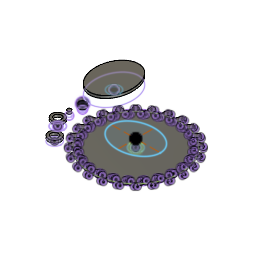
Duck Machine Gear 1 (Autodesk Fusion 360 design; units mm, degrees)
part number: 2026-02-17-17-01-41-865
Autodesk Fusion 360 part; units mm, degrees
(part 1 of 6)
sketch "Base Circle" plane through (0, 0, 0) normal (0, 0, 1) x (1, 0, 0)
  circle A0 centre (0, 0) radius 65.058
  circle A1 centre (0, 0) radius 2.45
extrude "Extrude3" add sketch "Base Circle" along normal blind 4.2 makes body 1
sketch "Gear Tooth" plane through (0, 0, 0) normal (0, 0, 1) x (1, 0, 0)
  spline S0 degree 5 poles (67.4396, -5.4307) (67.47, -5.4332) (67.531, -5.4373) (67.6225, -5.4412) (67.7446, -5.442) (67.8973, -5.437) (68.0502, -5.4277) (68.2031, -5.4157) (68.3561, -5.4023) (68.5091, -5.3879) (68.6621, -5.3725) (68.815, -5.3558) (68.968, -5.3372) (69.1209, -5.3166) (69.2738, -5.2939) (69.4267, -5.2693) (69.5795, -5.243) (69.7323, -5.2153) (69.885, -5.1864) (70.0377, -5.1565) (70.1903, -5.1253) (70.3428, -5.093) (70.4953, -5.0595) (70.6477, -5.0246) (70.8, -4.9885) (70.9522, -4.9511) (71.1044, -4.9126) (71.2565, -4.873) (71.4084, -4.8323) (71.5603, -4.7906) (71.7121, -4.7478) (71.8638, -4.704) (72.0153, -4.6592) (72.1668, -4.6134) (72.3182, -4.5666) (72.4695, -4.5187) (72.6206, -4.4699) (72.7716, -4.4202) (72.9226, -4.3695) (73.0734, -4.3179) (73.224, -4.2653) (73.3746, -4.2119) (73.525, -4.1576) (73.6753, -4.1023) (73.8255, -4.0462) (73.9756, -3.9892) (74.1255, -3.9313) (74.2752, -3.8726) (74.4249, -3.8131) (74.5744, -3.7527) (74.7237, -3.6914) (74.873, -3.6294) (75.022, -3.5665) (75.171, -3.5028) (75.3197, -3.4383) (75.4684, -3.373) (75.6168, -3.3069) (75.7652, -3.2401) (75.9133, -3.1724) (76.0614, -3.104) (76.2092, -3.0348) (76.3569, -2.9648) (76.5044, -2.8941) (76.6518, -2.8227) (76.799, -2.7505) (76.946, -2.6775) (77.0929, -2.6038) (77.2396, -2.5294) (77.3861, -2.4543) (77.5325, -2.3784) (77.6787, -2.3019) (77.7955, -2.24) (77.883, -2.1933) (77.9413, -2.1621) (77.9705, -2.1464) knots 0 0 0 0 0 0 0.01428571 0.02857143 0.04285714 0.05714286 0.07142857 0.08571429 0.1 0.11428571 0.12857143 0.14285714 0.15714286 0.17142857 0.18571429 0.2 0.21428571 0.22857143 0.24285714 0.25714286 0.27142857 0.28571429 0.3 0.31428571 0.32857143 0.34285714 0.35714286 0.37142857 0.38571429 0.4 0.41428571 0.42857143 0.44285714 0.45714286 0.47142857 0.48571429 0.5 0.51428571 0.52857143 0.54285714 0.55714286 0.57142857 0.58571429 0.6 0.61428571 0.62857143 0.64285714 0.65714286 0.67142857 0.68571429 0.7 0.71428571 0.72857143 0.74285714 0.75714286 0.77142857 0.78571429 0.8 0.81428571 0.82857143 0.84285714 0.85714286 0.87142857 0.88571429 0.9 0.91428571 0.92857143 0.94285714 0.95714286 0.97142857 0.98571429 1 1 1 1 1 1
  spline S1 degree 5 poles (67.4396, 5.4307) (67.47, 5.4332) (67.531, 5.4373) (67.6225, 5.4412) (67.7446, 5.442) (67.8973, 5.437) (68.0502, 5.4277) (68.2031, 5.4157) (68.3561, 5.4023) (68.5091, 5.3879) (68.6621, 5.3725) (68.815, 5.3558) (68.968, 5.3372) (69.1209, 5.3166) (69.2738, 5.2939) (69.4267, 5.2693) (69.5795, 5.243) (69.7323, 5.2153) (69.885, 5.1864) (70.0377, 5.1565) (70.1903, 5.1253) (70.3428, 5.093) (70.4953, 5.0595) (70.6477, 5.0246) (70.8, 4.9885) (70.9522, 4.9511) (71.1044, 4.9126) (71.2565, 4.873) (71.4084, 4.8323) (71.5603, 4.7906) (71.7121, 4.7478) (71.8638, 4.704) (72.0153, 4.6592) (72.1668, 4.6134) (72.3182, 4.5666) (72.4695, 4.5187) (72.6206, 4.4699) (72.7716, 4.4202) (72.9226, 4.3695) (73.0734, 4.3179) (73.224, 4.2653) (73.3746, 4.2119) (73.525, 4.1576) (73.6753, 4.1023) (73.8255, 4.0462) (73.9756, 3.9892) (74.1255, 3.9313) (74.2752, 3.8726) (74.4249, 3.8131) (74.5744, 3.7527) (74.7237, 3.6914) (74.873, 3.6294) (75.022, 3.5665) (75.171, 3.5028) (75.3197, 3.4383) (75.4684, 3.373) (75.6168, 3.3069) (75.7652, 3.2401) (75.9133, 3.1724) (76.0614, 3.104) (76.2092, 3.0348) (76.3569, 2.9648) (76.5044, 2.8941) (76.6518, 2.8227) (76.799, 2.7505) (76.946, 2.6775) (77.0929, 2.6038) (77.2396, 2.5294) (77.3861, 2.4543) (77.5325, 2.3784) (77.6787, 2.3019) (77.7955, 2.24) (77.883, 2.1933) (77.9413, 2.1621) (77.9705, 2.1464) knots 0 0 0 0 0 0 0.01428571 0.02857143 0.04285714 0.05714286 0.07142857 0.08571429 0.1 0.11428571 0.12857143 0.14285714 0.15714286 0.17142857 0.18571429 0.2 0.21428571 0.22857143 0.24285714 0.25714286 0.27142857 0.28571429 0.3 0.31428571 0.32857143 0.34285714 0.35714286 0.37142857 0.38571429 0.4 0.41428571 0.42857143 0.44285714 0.45714286 0.47142857 0.48571429 0.5 0.51428571 0.52857143 0.54285714 0.55714286 0.57142857 0.58571429 0.6 0.61428571 0.62857143 0.64285714 0.65714286 0.67142857 0.68571429 0.7 0.71428571 0.72857143 0.74285714 0.75714286 0.77142857 0.78571429 0.8 0.81428571 0.82857143 0.84285714 0.85714286 0.87142857 0.88571429 0.9 0.91428571 0.92857143 0.94285714 0.95714286 0.97142857 0.98571429 1 1 1 1 1 1
  arc A0 (77.9705, -2.1464) -> (77.9705, 2.1464) centre (0, 0) ccw
  line L0 (64.8381, -5.2213) -> (67.4396, -5.4307)
  line L1 (64.8381, 5.2213) -> (67.4396, 5.4307)
  line L2 (64.8381, -5.2213) -> (64.8381, 5.2213)
  point P0 (68.1817, -5.4171)
  point P1 (68.9286, -5.3417)
  point P2 (69.6784, -5.2249)
  point P3 (70.4303, -5.0736)
  point P4 (71.1836, -4.8918)
  point P5 (71.938, -4.682)
  point P6 (72.6931, -4.4459)
  point P7 (73.4485, -4.1851)
  point P8 (74.2039, -3.9005)
  point P9 (74.959, -3.5929)
  point P10 (75.7135, -3.2632)
  point P11 (76.4671, -2.9119)
  point P12 (77.2195, -2.5395)
  point P13 (68.1817, 5.4171)
  point P14 (68.9286, 5.3417)
  point P15 (69.6784, 5.2249)
  point P16 (70.4303, 5.0736)
  point P17 (71.1836, 4.8918)
  point P18 (71.938, 4.682)
  point P19 (72.6931, 4.4459)
  point P20 (73.4485, 4.1851)
  point P21 (74.2039, 3.9005)
  point P22 (74.959, 3.5929)
  point P23 (75.7135, 3.2632)
  point P24 (76.4671, 2.9119)
  point P25 (77.2195, 2.5395)
extrude "Extrude4" add sketch "Gear Tooth" along normal blind 4.2 bodies 1
fillet "Fillet2" radius 2 2 edges at (64.8481, -5.2221, 2.1) (64.8481, 5.2221, 2.1) on bodies 1
pattern_circular "C-Pattern2" count 24 over 360 about axis through (0, 0, 0) along (0, 0, 1) of "Extrude4", "Fillet2"
sketch "Diametrial Pitch Circle" plane through (0, 0, 0) normal (0, 0, 1) x (1, 0, 0)
  circle A0 centre (0, 0) radius 72 construction
sketch "Spacer and Cap" plane through (0, 0, 4.2) normal (0, 0, 1) x (-1, 0, 0)
  arc A0 (-64.3117, 9.8261) -> (-64.6635, 7.1538) centre (0, 0) ccw
  arc A1 (-66.8119, 5.3802) -> (-64.6635, 7.1538) centre (-66.6514, 7.3737) ccw
  line L0 (-66.8119, 5.3802) -> (-67.4396, 5.4307)
  spline S0 degree 5 poles (-67.4396, 5.4307) (-67.47, 5.4332) (-67.531, 5.4373) (-67.6225, 5.4412) (-67.7446, 5.442) (-67.8973, 5.437) (-68.0502, 5.4277) (-68.2031, 5.4157) (-68.3561, 5.4023) (-68.5091, 5.3879) (-68.6621, 5.3725) (-68.815, 5.3558) (-68.968, 5.3372) (-69.1209, 5.3166) (-69.2738, 5.2939) (-69.4267, 5.2693) (-69.5795, 5.243) (-69.7323, 5.2153) (-69.885, 5.1864) (-70.0377, 5.1565) (-70.1903, 5.1253) (-70.3428, 5.093) (-70.4953, 5.0595) (-70.6477, 5.0246) (-70.8, 4.9885) (-70.9522, 4.9511) (-71.1044, 4.9126) (-71.2565, 4.873) (-71.4084, 4.8323) (-71.5603, 4.7906) (-71.7121, 4.7478) (-71.8638, 4.704) (-72.0153, 4.6592) (-72.1668, 4.6134) (-72.3182, 4.5666) (-72.4695, 4.5187) (-72.6206, 4.4699) (-72.7716, 4.4202) (-72.9226, 4.3695) (-73.0734, 4.3179) (-73.224, 4.2653) (-73.3746, 4.2119) (-73.525, 4.1576) (-73.6753, 4.1023) (-73.8255, 4.0462) (-73.9756, 3.9892) (-74.1255, 3.9313) (-74.2752, 3.8726) (-74.4249, 3.8131) (-74.5744, 3.7527) (-74.7237, 3.6914) (-74.873, 3.6294) (-75.022, 3.5665) (-75.171, 3.5028) (-75.3197, 3.4383) (-75.4684, 3.373) (-75.6168, 3.3069) (-75.7652, 3.2401) (-75.9133, 3.1724) (-76.0614, 3.104) (-76.2092, 3.0348) (-76.3569, 2.9648) (-76.5044, 2.8941) (-76.6518, 2.8227) (-76.799, 2.7505) (-76.946, 2.6775) (-77.0929, 2.6038) (-77.2396, 2.5294) (-77.3861, 2.4543) (-77.5325, 2.3784) (-77.6787, 2.3019) (-77.7955, 2.24) (-77.883, 2.1933) (-77.9413, 2.1621) (-77.9705, 2.1464) knots 0 0 0 0 0 0 0.01428571 0.02857143 0.04285714 0.05714286 0.07142857 0.08571429 0.1 0.11428571 0.12857143 0.14285714 0.15714286 0.17142857 0.18571429 0.2 0.21428571 0.22857143 0.24285714 0.25714286 0.27142857 0.28571429 0.3 0.31428571 0.32857143 0.34285714 0.35714286 0.37142857 0.38571429 0.4 0.41428571 0.42857143 0.44285714 0.45714286 0.47142857 0.48571429 0.5 0.51428571 0.52857143 0.54285714 0.55714286 0.57142857 0.58571429 0.6 0.61428571 0.62857143 0.64285714 0.65714286 0.67142857 0.68571429 0.7 0.71428571 0.72857143 0.74285714 0.75714286 0.77142857 0.78571429 0.8 0.81428571 0.82857143 0.84285714 0.85714286 0.87142857 0.88571429 0.9 0.91428571 0.92857143 0.94285714 0.95714286 0.97142857 0.98571429 1 1 1 1 1 1
  arc A2 (-77.9705, 2.1464) -> (-77.9705, -2.1464) centre (0, 0) ccw
  spline S1 degree 5 poles (-77.9705, -2.1464) (-77.9413, -2.1621) (-77.883, -2.1933) (-77.7955, -2.24) (-77.6787, -2.3019) (-77.5325, -2.3784) (-77.3861, -2.4543) (-77.2396, -2.5294) (-77.0929, -2.6038) (-76.946, -2.6775) (-76.799, -2.7505) (-76.6518, -2.8227) (-76.5044, -2.8941) (-76.3569, -2.9648) (-76.2092, -3.0348) (-76.0614, -3.104) (-75.9133, -3.1724) (-75.7652, -3.2401) (-75.6168, -3.3069) (-75.4684, -3.373) (-75.3197, -3.4383) (-75.171, -3.5028) (-75.022, -3.5665) (-74.873, -3.6294) (-74.7237, -3.6914) (-74.5744, -3.7527) (-74.4249, -3.8131) (-74.2752, -3.8726) (-74.1255, -3.9313) (-73.9756, -3.9892) (-73.8255, -4.0462) (-73.6753, -4.1023) (-73.525, -4.1576) (-73.3746, -4.2119) (-73.224, -4.2653) (-73.0734, -4.3179) (-72.9226, -4.3695) (-72.7716, -4.4202) (-72.6206, -4.4699) (-72.4695, -4.5187) (-72.3182, -4.5666) (-72.1668, -4.6134) (-72.0153, -4.6592) (-71.8638, -4.704) (-71.7121, -4.7478) (-71.5603, -4.7906) (-71.4084, -4.8323) (-71.2565, -4.873) (-71.1044, -4.9126) (-70.9522, -4.9511) (-70.8, -4.9885) (-70.6477, -5.0246) (-70.4953, -5.0595) (-70.3428, -5.093) (-70.1903, -5.1253) (-70.0377, -5.1565) (-69.885, -5.1864) (-69.7323, -5.2153) (-69.5795, -5.243) (-69.4267, -5.2693) (-69.2738, -5.2939) (-69.1209, -5.3166) (-68.968, -5.3372) (-68.815, -5.3558) (-68.6621, -5.3725) (-68.5091, -5.3879) (-68.3561, -5.4023) (-68.2031, -5.4157) (-68.0502, -5.4277) (-67.8973, -5.437) (-67.7446, -5.442) (-67.6225, -5.4412) (-67.531, -5.4373) (-67.47, -5.4332) (-67.4396, -5.4307) knots -1 -1 -1 -1 -1 -1 -0.98571429 -0.97142857 -0.95714286 -0.94285714 -0.92857143 -0.91428571 -0.9 -0.88571429 -0.87142857 -0.85714286 -0.84285714 -0.82857143 -0.81428571 -0.8 -0.78571429 -0.77142857 -0.75714286 -0.74285714 -0.72857143 -0.71428571 -0.7 -0.68571429 -0.67142857 -0.65714286 -0.64285714 -0.62857143 -0.61428571 -0.6 -0.58571429 -0.57142857 -0.55714286 -0.54285714 -0.52857143 -0.51428571 -0.5 -0.48571429 -0.47142857 -0.45714286 -0.44285714 -0.42857143 -0.41428571 -0.4 -0.38571429 -0.37142857 -0.35714286 -0.34285714 -0.32857143 -0.31428571 -0.3 -0.28571429 -0.27142857 -0.25714286 -0.24285714 -0.22857143 -0.21428571 -0.2 -0.18571429 -0.17142857 -0.15714286 -0.14285714 -0.12857143 -0.11428571 -0.1 -0.08571429 -0.07142857 -0.05714286 -0.04285714 -0.02857143 -0.01428571 0 0 0 0 0 0
  line L1 (-67.4396, -5.4307) -> (-66.8119, -5.3802)
  arc A3 (-64.6635, -7.1538) -> (-66.8119, -5.3802) centre (-66.6514, -7.3737) ccw
  arc A4 (-64.6635, -7.1538) -> (-64.3117, -9.8261) centre (0, 0) ccw
  arc A5 (-65.9278, -12.0953) -> (-64.3117, -9.8261) centre (-66.2887, -10.1281) ccw
  line L2 (-65.9278, -12.0953) -> (-66.5472, -12.2089)
  spline S2 degree 5 poles (-66.5472, -12.2089) (-66.5773, -12.2145) (-66.6372, -12.2262) (-66.7266, -12.2462) (-66.8447, -12.277) (-66.991, -12.3214) (-67.1362, -12.37) (-67.2808, -12.4211) (-67.4251, -12.4737) (-67.5692, -12.5271) (-67.713, -12.5816) (-67.8564, -12.6374) (-67.9993, -12.6949) (-68.1417, -12.7544) (-68.2835, -12.8159) (-68.4248, -12.8792) (-68.5656, -12.9442) (-68.7061, -13.0105) (-68.8461, -13.0779) (-68.9858, -13.1463) (-69.1252, -13.2159) (-69.2641, -13.2866) (-69.4027, -13.3585) (-69.5409, -13.4316) (-69.6787, -13.5059) (-69.816, -13.5814) (-69.953, -13.658) (-70.0897, -13.7356) (-70.2259, -13.8142) (-70.3618, -13.8938) (-70.4974, -13.9744) (-70.6326, -14.056) (-70.7674, -14.1385) (-70.9018, -14.2219) (-71.0359, -14.3063) (-71.1697, -14.3917) (-71.303, -14.478) (-71.436, -14.5651) (-71.5687, -14.6531) (-71.701, -14.742) (-71.8329, -14.8318) (-71.9645, -14.9224) (-72.0958, -15.0138) (-72.2267, -15.106) (-72.3572, -15.1991) (-72.4874, -15.293) (-72.6172, -15.3877) (-72.7467, -15.4832) (-72.8758, -15.5794) (-73.0046, -15.6765) (-73.133, -15.7743) (-73.2611, -15.8729) (-73.3888, -15.9722) (-73.5162, -16.0722) (-73.6432, -16.173) (-73.7698, -16.2746) (-73.8962, -16.3768) (-74.0221, -16.4798) (-74.1477, -16.5835) (-74.273, -16.6879) (-74.3979, -16.793) (-74.5225, -16.8988) (-74.6467, -17.0053) (-74.7705, -17.1124) (-74.894, -17.2203) (-75.0172, -17.3288) (-75.14, -17.438) (-75.2624, -17.5478) (-75.3845, -17.6583) (-75.5062, -17.7695) (-75.6276, -17.8813) (-75.7244, -17.9712) (-75.7969, -18.039) (-75.8451, -18.0843) (-75.8692, -18.107) knots 0 0 0 0 0 0 0.01428571 0.02857143 0.04285714 0.05714286 0.07142857 0.08571429 0.1 0.11428571 0.12857143 0.14285714 0.15714286 0.17142857 0.18571429 0.2 0.21428571 0.22857143 0.24285714 0.25714286 0.27142857 0.28571429 0.3 0.31428571 0.32857143 0.34285714 0.35714286 0.37142857 0.38571429 0.4 0.41428571 0.42857143 0.44285714 0.45714286 0.47142857 0.48571429 0.5 0.51428571 0.52857143 0.54285714 0.55714286 0.57142857 0.58571429 0.6 0.61428571 0.62857143 0.64285714 0.65714286 0.67142857 0.68571429 0.7 0.71428571 0.72857143 0.74285714 0.75714286 0.77142857 0.78571429 0.8 0.81428571 0.82857143 0.84285714 0.85714286 0.87142857 0.88571429 0.9 0.91428571 0.92857143 0.94285714 0.95714286 0.97142857 0.98571429 1 1 1 1 1 1
  arc A6 (-75.8692, -18.107) -> (-74.7582, -22.2535) centre (0, 0) ccw
  spline S3 degree 5 poles (-74.7582, -22.2535) (-74.7259, -22.2611) (-74.6615, -22.2762) (-74.5649, -22.2987) (-74.4361, -22.3281) (-74.275, -22.3643) (-74.1141, -22.3997) (-73.9531, -22.4343) (-73.7921, -22.4682) (-73.6312, -22.5014) (-73.4703, -22.5338) (-73.3094, -22.5654) (-73.1486, -22.5963) (-72.9877, -22.6264) (-72.827, -22.6558) (-72.6663, -22.6843) (-72.5056, -22.7121) (-72.3449, -22.7391) (-72.1844, -22.7653) (-72.0239, -22.7907) (-71.8634, -22.8153) (-71.703, -22.8391) (-71.5426, -22.8621) (-71.3824, -22.8842) (-71.2222, -22.9056) (-71.0621, -22.9261) (-70.902, -22.9457) (-70.7421, -22.9645) (-70.5822, -22.9825) (-70.4224, -22.9996) (-70.2627, -23.0158) (-70.1031, -23.0311) (-69.9437, -23.0456) (-69.7843, -23.0591) (-69.625, -23.0718) (-69.4659, -23.0835) (-69.3069, -23.0944) (-69.148, -23.1043) (-68.9892, -23.1132) (-68.8306, -23.1213) (-68.6721, -23.1283) (-68.5138, -23.1344) (-68.3556, -23.1394) (-68.1976, -23.1435) (-68.0397, -23.1465) (-67.8821, -23.1485) (-67.7246, -23.1495) (-67.5672, -23.1494) (-67.4101, -23.1484) (-67.2532, -23.1462) (-67.0965, -23.1429) (-66.94, -23.1384) (-66.7838, -23.1326) (-66.6278, -23.1256) (-66.4721, -23.1173) (-66.3166, -23.1078) (-66.1614, -23.0973) (-66.0064, -23.0856) (-65.8517, -23.0728) (-65.6973, -23.0587) (-65.5432, -23.0429) (-65.3896, -23.0253) (-65.2366, -23.0056) (-65.084, -22.9839) (-64.9319, -22.9605) (-64.7802, -22.9358) (-64.6287, -22.91) (-64.4775, -22.8834) (-64.3267, -22.8554) (-64.1766, -22.8249) (-64.0277, -22.7902) (-63.91, -22.7578) (-63.8226, -22.7304) (-63.7648, -22.7106) (-63.736, -22.7003) knots -1 -1 -1 -1 -1 -1 -0.98571429 -0.97142857 -0.95714286 -0.94285714 -0.92857143 -0.91428571 -0.9 -0.88571429 -0.87142857 -0.85714286 -0.84285714 -0.82857143 -0.81428571 -0.8 -0.78571429 -0.77142857 -0.75714286 -0.74285714 -0.72857143 -0.71428571 -0.7 -0.68571429 -0.67142857 -0.65714286 -0.64285714 -0.62857143 -0.61428571 -0.6 -0.58571429 -0.57142857 -0.55714286 -0.54285714 -0.52857143 -0.51428571 -0.5 -0.48571429 -0.47142857 -0.45714286 -0.44285714 -0.42857143 -0.41428571 -0.4 -0.38571429 -0.37142857 -0.35714286 -0.34285714 -0.32857143 -0.31428571 -0.3 -0.28571429 -0.27142857 -0.25714286 -0.24285714 -0.22857143 -0.21428571 -0.2 -0.18571429 -0.17142857 -0.15714286 -0.14285714 -0.12857143 -0.11428571 -0.1 -0.08571429 -0.07142857 -0.05714286 -0.04285714 -0.02857143 -0.01428571 0 0 0 0 0 0
  line L3 (-63.736, -22.7003) -> (-63.1428, -22.4891)
  arc A7 (-60.6086, -23.6462) -> (-63.1428, -22.4891) centre (-62.4718, -24.3731) ccw
  arc A8 (-60.6086, -23.6462) -> (-59.5771, -26.1363) centre (0, 0) ccw
  arc A9 (-60.5509, -28.7466) -> (-59.5771, -26.1363) centre (-61.4086, -26.9398) ccw
  line L4 (-60.5509, -28.7466) -> (-61.1197, -29.0166)
  spline S4 degree 5 poles (-61.1197, -29.0166) (-61.1474, -29.0297) (-61.2022, -29.0566) (-61.2834, -29.099) (-61.3895, -29.1594) (-61.5193, -29.2401) (-61.647, -29.3246) (-61.7735, -29.4115) (-61.8992, -29.4995) (-62.0245, -29.5885) (-62.1493, -29.6783) (-62.2734, -29.7693) (-62.3966, -29.8618) (-62.5188, -29.9561) (-62.6398, -30.0523) (-62.7599, -30.15) (-62.8791, -30.2492) (-62.9976, -30.3496) (-63.1154, -30.4509) (-63.2327, -30.5532) (-63.3493, -30.6565) (-63.4652, -30.7607) (-63.5805, -30.866) (-63.695, -30.9724) (-63.8088, -31.0799) (-63.922, -31.1883) (-64.0345, -31.2978) (-64.1464, -31.4081) (-64.2576, -31.5193) (-64.3683, -31.6314) (-64.4784, -31.7443) (-64.5879, -31.8581) (-64.6967, -31.9727) (-64.805, -32.0881) (-64.9127, -32.2043) (-65.0198, -32.3214) (-65.1263, -32.4392) (-65.2322, -32.5578) (-65.3375, -32.6772) (-65.4423, -32.7973) (-65.5465, -32.9181) (-65.6502, -33.0397) (-65.7533, -33.162) (-65.8559, -33.2849) (-65.9579, -33.4086) (-66.0593, -33.533) (-66.1602, -33.6581) (-66.2606, -33.7838) (-66.3604, -33.9102) (-66.4596, -34.0373) (-66.5584, -34.165) (-66.6566, -34.2934) (-66.7542, -34.4224) (-66.8514, -34.552) (-66.948, -34.6822) (-67.044, -34.8131) (-67.1396, -34.9445) (-67.2346, -35.0766) (-67.3291, -35.2093) (-67.4231, -35.3425) (-67.5165, -35.4764) (-67.6094, -35.6108) (-67.7019, -35.7458) (-67.7938, -35.8814) (-67.8851, -36.0175) (-67.976, -36.1542) (-68.0663, -36.2915) (-68.1562, -36.4293) (-68.2455, -36.5676) (-68.3343, -36.7065) (-68.4226, -36.8459) (-68.4929, -36.9578) (-68.5453, -37.042) (-68.5802, -37.0983) (-68.5976, -37.1264) knots 0 0 0 0 0 0 0.01428571 0.02857143 0.04285714 0.05714286 0.07142857 0.08571429 0.1 0.11428571 0.12857143 0.14285714 0.15714286 0.17142857 0.18571429 0.2 0.21428571 0.22857143 0.24285714 0.25714286 0.27142857 0.28571429 0.3 0.31428571 0.32857143 0.34285714 0.35714286 0.37142857 0.38571429 0.4 0.41428571 0.42857143 0.44285714 0.45714286 0.47142857 0.48571429 0.5 0.51428571 0.52857143 0.54285714 0.55714286 0.57142857 0.58571429 0.6 0.61428571 0.62857143 0.64285714 0.65714286 0.67142857 0.68571429 0.7 0.71428571 0.72857143 0.74285714 0.75714286 0.77142857 0.78571429 0.8 0.81428571 0.82857143 0.84285714 0.85714286 0.87142857 0.88571429 0.9 0.91428571 0.92857143 0.94285714 0.95714286 0.97142857 0.98571429 1 1 1 1 1 1
  arc A10 (-68.5976, -37.1264) -> (-66.4512, -40.8441) centre (0, 0) ccw
  spline S5 degree 5 poles (-66.4512, -40.8441) (-66.4181, -40.8431) (-66.352, -40.841) (-66.2528, -40.8377) (-66.1208, -40.8328) (-65.9559, -40.826) (-65.7912, -40.8186) (-65.6268, -40.8104) (-65.4625, -40.8015) (-65.2985, -40.7918) (-65.1347, -40.7815) (-64.9711, -40.7704) (-64.8077, -40.7586) (-64.6446, -40.7461) (-64.4817, -40.7328) (-64.3191, -40.7188) (-64.1567, -40.7041) (-63.9945, -40.6886) (-63.8327, -40.6723) (-63.671, -40.6553) (-63.5097, -40.6375) (-63.3486, -40.619) (-63.1877, -40.5997) (-63.0272, -40.5796) (-62.867, -40.5587) (-62.707, -40.5371) (-62.5473, -40.5146) (-62.3879, -40.4914) (-62.2289, -40.4674) (-62.0701, -40.4425) (-61.9117, -40.4169) (-61.7535, -40.3904) (-61.5958, -40.3631) (-61.4383, -40.3349) (-61.2812, -40.3059) (-61.1244, -40.2761) (-60.968, -40.2454) (-60.812, -40.2138) (-60.6563, -40.1814) (-60.501, -40.1481) (-60.3461, -40.1139) (-60.1916, -40.0787) (-60.0375, -40.0427) (-59.8838, -40.0057) (-59.7306, -39.9678) (-59.5778, -39.9289) (-59.4254, -39.8891) (-59.2734, -39.8483) (-59.1219, -39.8066) (-58.9709, -39.7639) (-58.8204, -39.7201) (-58.6704, -39.6753) (-58.521, -39.6293) (-58.3722, -39.5821) (-58.2239, -39.5338) (-58.0762, -39.4845) (-57.929, -39.4341) (-57.7823, -39.3827) (-57.6362, -39.3303) (-57.4907, -39.2767) (-57.346, -39.2216) (-57.2022, -39.1648) (-57.0594, -39.1062) (-56.9177, -39.0457) (-56.7768, -38.9838) (-56.6367, -38.9206) (-56.497, -38.8565) (-56.3578, -38.7917) (-56.2194, -38.7256) (-56.0823, -38.6572) (-55.9475, -38.5852) (-55.8422, -38.5235) (-55.7649, -38.4744) (-55.7142, -38.4403) (-55.689, -38.4229) knots -1 -1 -1 -1 -1 -1 -0.98571429 -0.97142857 -0.95714286 -0.94285714 -0.92857143 -0.91428571 -0.9 -0.88571429 -0.87142857 -0.85714286 -0.84285714 -0.82857143 -0.81428571 -0.8 -0.78571429 -0.77142857 -0.75714286 -0.74285714 -0.72857143 -0.71428571 -0.7 -0.68571429 -0.67142857 -0.65714286 -0.64285714 -0.62857143 -0.61428571 -0.6 -0.58571429 -0.57142857 -0.55714286 -0.54285714 -0.52857143 -0.51428571 -0.5 -0.48571429 -0.47142857 -0.45714286 -0.44285714 -0.42857143 -0.41428571 -0.4 -0.38571429 -0.37142857 -0.35714286 -0.34285714 -0.32857143 -0.31428571 -0.3 -0.28571429 -0.27142857 -0.25714286 -0.24285714 -0.22857143 -0.21428571 -0.2 -0.18571429 -0.17142857 -0.15714286 -0.14285714 -0.12857143 -0.11428571 -0.1 -0.08571429 -0.07142857 -0.05714286 -0.04285714 -0.02857143 -0.01428571 0 0 0 0 0 0
  line L5 (-55.689, -38.4229) -> (-55.1707, -38.0653)
  arc A11 (-52.4233, -38.5271) -> (-55.1707, -38.0653) centre (-54.0349, -39.7115) ccw
  arc A12 (-52.4233, -38.5271) -> (-50.7825, -40.6655) centre (0, 0) ccw
  arc A13 (-51.0475, -43.4388) -> (-50.7825, -40.6655) centre (-52.3437, -41.9156) ccw
  line L6 (-51.0475, -43.4388) -> (-51.5271, -43.8469)
  spline S6 degree 5 poles (-51.5271, -43.8469) (-51.5504, -43.8667) (-51.5964, -43.9068) (-51.6639, -43.9688) (-51.7507, -44.0546) (-51.8552, -44.1661) (-51.9567, -44.2808) (-52.0564, -44.3974) (-52.155, -44.5151) (-52.253, -44.6334) (-52.3503, -44.7525) (-52.4467, -44.8725) (-52.5417, -44.9937) (-52.6353, -45.1165) (-52.7273, -45.2406) (-52.818, -45.3662) (-52.9075, -45.4928) (-52.996, -45.6204) (-53.0835, -45.7488) (-53.1703, -45.878) (-53.2562, -46.0079) (-53.3412, -46.1386) (-53.4253, -46.2701) (-53.5084, -46.4025) (-53.5905, -46.5358) (-53.6718, -46.6699) (-53.7521, -46.8047) (-53.8316, -46.9402) (-53.9103, -47.0764) (-53.9882, -47.2133) (-54.0653, -47.3509) (-54.1416, -47.4891) (-54.2171, -47.628) (-54.2918, -47.7675) (-54.3657, -47.9076) (-54.4389, -48.0484) (-54.5112, -48.1898) (-54.5829, -48.3318) (-54.6537, -48.4743) (-54.7239, -48.6175) (-54.7933, -48.7612) (-54.8619, -48.9054) (-54.9299, -49.0502) (-54.9971, -49.1955) (-55.0636, -49.3414) (-55.1294, -49.4878) (-55.1945, -49.6347) (-55.2589, -49.7822) (-55.3226, -49.9301) (-55.3856, -50.0785) (-55.4479, -50.2274) (-55.5095, -50.3768) (-55.5705, -50.5267) (-55.6307, -50.677) (-55.6903, -50.8279) (-55.7493, -50.9791) (-55.8075, -51.1308) (-55.8651, -51.283) (-55.9221, -51.4356) (-55.9783, -51.5886) (-56.034, -51.7421) (-56.0889, -51.896) (-56.1433, -52.0503) (-56.1969, -52.2051) (-56.25, -52.3602) (-56.3024, -52.5158) (-56.3541, -52.6717) (-56.4052, -52.8281) (-56.4557, -52.9848) (-56.5056, -53.1419) (-56.5548, -53.2995) (-56.5936, -53.4258) (-56.6225, -53.5207) (-56.6416, -53.584) (-56.6512, -53.6157) knots 0 0 0 0 0 0 0.01428571 0.02857143 0.04285714 0.05714286 0.07142857 0.08571429 0.1 0.11428571 0.12857143 0.14285714 0.15714286 0.17142857 0.18571429 0.2 0.21428571 0.22857143 0.24285714 0.25714286 0.27142857 0.28571429 0.3 0.31428571 0.32857143 0.34285714 0.35714286 0.37142857 0.38571429 0.4 0.41428571 0.42857143 0.44285714 0.45714286 0.47142857 0.48571429 0.5 0.51428571 0.52857143 0.54285714 0.55714286 0.57142857 0.58571429 0.6 0.61428571 0.62857143 0.64285714 0.65714286 0.67142857 0.68571429 0.7 0.71428571 0.72857143 0.74285714 0.75714286 0.77142857 0.78571429 0.8 0.81428571 0.82857143 0.84285714 0.85714286 0.87142857 0.88571429 0.9 0.91428571 0.92857143 0.94285714 0.95714286 0.97142857 0.98571429 1 1 1 1 1 1
  arc A14 (-56.6512, -53.6157) -> (-53.6157, -56.6512) centre (0, 0) ccw
  spline S7 degree 5 poles (-53.6157, -56.6512) (-53.584, -56.6416) (-53.5207, -56.6225) (-53.4258, -56.5936) (-53.2995, -56.5548) (-53.1419, -56.5056) (-52.9848, -56.4557) (-52.8281, -56.4052) (-52.6717, -56.3541) (-52.5158, -56.3024) (-52.3602, -56.25) (-52.2051, -56.1969) (-52.0503, -56.1433) (-51.896, -56.0889) (-51.7421, -56.034) (-51.5886, -55.9783) (-51.4356, -55.9221) (-51.283, -55.8651) (-51.1308, -55.8075) (-50.9791, -55.7493) (-50.8279, -55.6903) (-50.677, -55.6307) (-50.5267, -55.5705) (-50.3768, -55.5095) (-50.2274, -55.4479) (-50.0785, -55.3856) (-49.9301, -55.3226) (-49.7822, -55.2589) (-49.6347, -55.1945) (-49.4878, -55.1294) (-49.3414, -55.0636) (-49.1955, -54.9971) (-49.0502, -54.9299) (-48.9054, -54.8619) (-48.7612, -54.7933) (-48.6175, -54.7239) (-48.4743, -54.6537) (-48.3318, -54.5829) (-48.1898, -54.5112) (-48.0484, -54.4389) (-47.9076, -54.3657) (-47.7675, -54.2918) (-47.628, -54.2171) (-47.4891, -54.1416) (-47.3509, -54.0653) (-47.2133, -53.9882) (-47.0764, -53.9103) (-46.9402, -53.8316) (-46.8047, -53.7521) (-46.6699, -53.6718) (-46.5358, -53.5905) (-46.4025, -53.5084) (-46.2701, -53.4253) (-46.1386, -53.3412) (-46.0079, -53.2562) (-45.878, -53.1703) (-45.7488, -53.0835) (-45.6204, -52.996) (-45.4928, -52.9075) (-45.3662, -52.818) (-45.2406, -52.7273) (-45.1165, -52.6353) (-44.9937, -52.5417) (-44.8725, -52.4467) (-44.7525, -52.3503) (-44.6334, -52.253) (-44.5151, -52.155) (-44.3974, -52.0564) (-44.2808, -51.9567) (-44.1661, -51.8552) (-44.0546, -51.7507) (-43.9688, -51.6639) (-43.9068, -51.5964) (-43.8667, -51.5504) (-43.8469, -51.5271) knots -1 -1 -1 -1 -1 -1 -0.98571429 -0.97142857 -0.95714286 -0.94285714 -0.92857143 -0.91428571 -0.9 -0.88571429 -0.87142857 -0.85714286 -0.84285714 -0.82857143 -0.81428571 -0.8 -0.78571429 -0.77142857 -0.75714286 -0.74285714 -0.72857143 -0.71428571 -0.7 -0.68571429 -0.67142857 -0.65714286 -0.64285714 -0.62857143 -0.61428571 -0.6 -0.58571429 -0.57142857 -0.55714286 -0.54285714 -0.52857143 -0.51428571 -0.5 -0.48571429 -0.47142857 -0.45714286 -0.44285714 -0.42857143 -0.41428571 -0.4 -0.38571429 -0.37142857 -0.35714286 -0.34285714 -0.32857143 -0.31428571 -0.3 -0.28571429 -0.27142857 -0.25714286 -0.24285714 -0.22857143 -0.21428571 -0.2 -0.18571429 -0.17142857 -0.15714286 -0.14285714 -0.12857143 -0.11428571 -0.1 -0.08571429 -0.07142857 -0.05714286 -0.04285714 -0.02857143 -0.01428571 0 0 0 0 0 0
  line L7 (-43.8469, -51.5271) -> (-43.4388, -51.0475)
  arc A15 (-40.6655, -50.7825) -> (-43.4388, -51.0475) centre (-41.9156, -52.3437) ccw
  arc A16 (-40.6655, -50.7825) -> (-38.5271, -52.4233) centre (0, 0) ccw
  arc A17 (-38.0653, -55.1707) -> (-38.5271, -52.4233) centre (-39.7115, -54.0349) ccw
  line L8 (-38.0653, -55.1707) -> (-38.4229, -55.689)
  spline S8 degree 5 poles (-38.4229, -55.689) (-38.4403, -55.7142) (-38.4744, -55.7649) (-38.5235, -55.8422) (-38.5852, -55.9475) (-38.6572, -56.0823) (-38.7256, -56.2194) (-38.7917, -56.3578) (-38.8565, -56.497) (-38.9206, -56.6367) (-38.9838, -56.7768) (-39.0457, -56.9177) (-39.1062, -57.0594) (-39.1648, -57.2022) (-39.2216, -57.346) (-39.2767, -57.4907) (-39.3303, -57.6362) (-39.3827, -57.7823) (-39.4341, -57.929) (-39.4845, -58.0762) (-39.5338, -58.2239) (-39.5821, -58.3722) (-39.6293, -58.521) (-39.6753, -58.6704) (-39.7201, -58.8204) (-39.7639, -58.9709) (-39.8066, -59.1219) (-39.8483, -59.2734) (-39.8891, -59.4254) (-39.9289, -59.5778) (-39.9678, -59.7306) (-40.0057, -59.8838) (-40.0427, -60.0375) (-40.0787, -60.1916) (-40.1139, -60.3461) (-40.1481, -60.501) (-40.1814, -60.6563) (-40.2138, -60.812) (-40.2454, -60.968) (-40.2761, -61.1244) (-40.3059, -61.2812) (-40.3349, -61.4383) (-40.3631, -61.5958) (-40.3904, -61.7535) (-40.4169, -61.9117) (-40.4425, -62.0701) (-40.4674, -62.2289) (-40.4914, -62.3879) (-40.5146, -62.5473) (-40.5371, -62.707) (-40.5587, -62.867) (-40.5796, -63.0272) (-40.5997, -63.1877) (-40.619, -63.3486) (-40.6375, -63.5097) (-40.6553, -63.671) (-40.6723, -63.8327) (-40.6886, -63.9945) (-40.7041, -64.1567) (-40.7188, -64.3191) (-40.7328, -64.4817) (-40.7461, -64.6446) (-40.7586, -64.8077) (-40.7704, -64.9711) (-40.7815, -65.1347) (-40.7918, -65.2985) (-40.8015, -65.4625) (-40.8104, -65.6268) (-40.8186, -65.7912) (-40.826, -65.9559) (-40.8328, -66.1208) (-40.8377, -66.2528) (-40.841, -66.352) (-40.8431, -66.4181) (-40.8441, -66.4512) knots 0 0 0 0 0 0 0.01428571 0.02857143 0.04285714 0.05714286 0.07142857 0.08571429 0.1 0.11428571 0.12857143 0.14285714 0.15714286 0.17142857 0.18571429 0.2 0.21428571 0.22857143 0.24285714 0.25714286 0.27142857 0.28571429 0.3 0.31428571 0.32857143 0.34285714 0.35714286 0.37142857 0.38571429 0.4 0.41428571 0.42857143 0.44285714 0.45714286 0.47142857 0.48571429 0.5 0.51428571 0.52857143 0.54285714 0.55714286 0.57142857 0.58571429 0.6 0.61428571 0.62857143 0.64285714 0.65714286 0.67142857 0.68571429 0.7 0.71428571 0.72857143 0.74285714 0.75714286 0.77142857 0.78571429 0.8 0.81428571 0.82857143 0.84285714 0.85714286 0.87142857 0.88571429 0.9 0.91428571 0.92857143 0.94285714 0.95714286 0.97142857 0.98571429 1 1 1 1 1 1
  arc A18 (-40.8441, -66.4512) -> (-37.1264, -68.5976) centre (0, 0) ccw
  spline S9 degree 5 poles (-37.1264, -68.5976) (-37.0983, -68.5802) (-37.042, -68.5453) (-36.9578, -68.4929) (-36.8459, -68.4226) (-36.7065, -68.3343) (-36.5676, -68.2455) (-36.4293, -68.1562) (-36.2915, -68.0663) (-36.1542, -67.976) (-36.0175, -67.8851) (-35.8814, -67.7938) (-35.7458, -67.7019) (-35.6108, -67.6094) (-35.4764, -67.5165) (-35.3425, -67.4231) (-35.2093, -67.3291) (-35.0766, -67.2346) (-34.9445, -67.1396) (-34.8131, -67.044) (-34.6822, -66.948) (-34.552, -66.8514) (-34.4224, -66.7542) (-34.2934, -66.6566) (-34.165, -66.5584) (-34.0373, -66.4596) (-33.9102, -66.3604) (-33.7838, -66.2606) (-33.6581, -66.1602) (-33.533, -66.0593) (-33.4086, -65.9579) (-33.2849, -65.8559) (-33.162, -65.7533) (-33.0397, -65.6502) (-32.9181, -65.5465) (-32.7973, -65.4423) (-32.6772, -65.3375) (-32.5578, -65.2322) (-32.4392, -65.1263) (-32.3214, -65.0198) (-32.2043, -64.9127) (-32.0881, -64.805) (-31.9727, -64.6967) (-31.8581, -64.5879) (-31.7443, -64.4784) (-31.6314, -64.3683) (-31.5193, -64.2576) (-31.4081, -64.1464) (-31.2978, -64.0345) (-31.1883, -63.922) (-31.0799, -63.8088) (-30.9724, -63.695) (-30.866, -63.5805) (-30.7607, -63.4652) (-30.6565, -63.3493) (-30.5532, -63.2327) (-30.4509, -63.1154) (-30.3496, -62.9976) (-30.2492, -62.8791) (-30.15, -62.7599) (-30.0523, -62.6398) (-29.9561, -62.5188) (-29.8618, -62.3966) (-29.7693, -62.2734) (-29.6783, -62.1493) (-29.5885, -62.0245) (-29.4995, -61.8992) (-29.4115, -61.7735) (-29.3246, -61.647) (-29.2401, -61.5193) (-29.1594, -61.3895) (-29.099, -61.2834) (-29.0566, -61.2022) (-29.0297, -61.1474) (-29.0166, -61.1197) knots -1 -1 -1 -1 -1 -1 -0.98571429 -0.97142857 -0.95714286 -0.94285714 -0.92857143 -0.91428571 -0.9 -0.88571429 -0.87142857 -0.85714286 -0.84285714 -0.82857143 -0.81428571 -0.8 -0.78571429 -0.77142857 -0.75714286 -0.74285714 -0.72857143 -0.71428571 -0.7 -0.68571429 -0.67142857 -0.65714286 -0.64285714 -0.62857143 -0.61428571 -0.6 -0.58571429 -0.57142857 -0.55714286 -0.54285714 -0.52857143 -0.51428571 -0.5 -0.48571429 -0.47142857 -0.45714286 -0.44285714 -0.42857143 -0.41428571 -0.4 -0.38571429 -0.37142857 -0.35714286 -0.34285714 -0.32857143 -0.31428571 -0.3 -0.28571429 -0.27142857 -0.25714286 -0.24285714 -0.22857143 -0.21428571 -0.2 -0.18571429 -0.17142857 -0.15714286 -0.14285714 -0.12857143 -0.11428571 -0.1 -0.08571429 -0.07142857 -0.05714286 -0.04285714 -0.02857143 -0.01428571 0 0 0 0 0 0
  line L9 (-29.0166, -61.1197) -> (-28.7466, -60.5509)
  arc A19 (-26.1363, -59.5771) -> (-28.7466, -60.5509) centre (-26.9398, -61.4086) ccw
  arc A20 (-26.1363, -59.5771) -> (-23.6462, -60.6086) centre (0, 0) ccw
  arc A21 (-22.4891, -63.1428) -> (-23.6462, -60.6086) centre (-24.3731, -62.4718) ccw
  line L10 (-22.4891, -63.1428) -> (-22.7003, -63.736)
  spline S10 degree 5 poles (-22.7003, -63.736) (-22.7106, -63.7648) (-22.7304, -63.8226) (-22.7578, -63.91) (-22.7902, -64.0277) (-22.8249, -64.1766) (-22.8554, -64.3267) (-22.8834, -64.4775) (-22.91, -64.6287) (-22.9358, -64.7802) (-22.9605, -64.9319) (-22.9839, -65.084) (-23.0056, -65.2366) (-23.0253, -65.3896) (-23.0429, -65.5432) (-23.0587, -65.6973) (-23.0728, -65.8517) (-23.0856, -66.0064) (-23.0973, -66.1614) (-23.1078, -66.3166) (-23.1173, -66.4721) (-23.1256, -66.6278) (-23.1326, -66.7838) (-23.1384, -66.94) (-23.1429, -67.0965) (-23.1462, -67.2532) (-23.1484, -67.4101) (-23.1494, -67.5672) (-23.1495, -67.7246) (-23.1485, -67.8821) (-23.1465, -68.0397) (-23.1435, -68.1976) (-23.1394, -68.3556) (-23.1344, -68.5138) (-23.1283, -68.6721) (-23.1213, -68.8306) (-23.1132, -68.9892) (-23.1043, -69.148) (-23.0944, -69.3069) (-23.0835, -69.4659) (-23.0718, -69.625) (-23.0591, -69.7843) (-23.0456, -69.9437) (-23.0311, -70.1031) (-23.0158, -70.2627) (-22.9996, -70.4224) (-22.9825, -70.5822) (-22.9645, -70.7421) (-22.9457, -70.902) (-22.9261, -71.0621) (-22.9056, -71.2222) (-22.8842, -71.3824) (-22.8621, -71.5426) (-22.8391, -71.703) (-22.8153, -71.8634) (-22.7907, -72.0239) (-22.7653, -72.1844) (-22.7391, -72.3449) (-22.7121, -72.5056) (-22.6843, -72.6663) (-22.6558, -72.827) (-22.6264, -72.9877) (-22.5963, -73.1486) (-22.5654, -73.3094) (-22.5338, -73.4703) (-22.5014, -73.6312) (-22.4682, -73.7921) (-22.4343, -73.9531) (-22.3997, -74.1141) (-22.3643, -74.275) (-22.3281, -74.4361) (-22.2987, -74.5649) (-22.2762, -74.6615) (-22.2611, -74.7259) (-22.2535, -74.7582) knots 0 0 0 0 0 0 0.01428571 0.02857143 0.04285714 0.05714286 0.07142857 0.08571429 0.1 0.11428571 0.12857143 0.14285714 0.15714286 0.17142857 0.18571429 0.2 0.21428571 0.22857143 0.24285714 0.25714286 0.27142857 0.28571429 0.3 0.31428571 0.32857143 0.34285714 0.35714286 0.37142857 0.38571429 0.4 0.41428571 0.42857143 0.44285714 0.45714286 0.47142857 0.48571429 0.5 0.51428571 0.52857143 0.54285714 0.55714286 0.57142857 0.58571429 0.6 0.61428571 0.62857143 0.64285714 0.65714286 0.67142857 0.68571429 0.7 0.71428571 0.72857143 0.74285714 0.75714286 0.77142857 0.78571429 0.8 0.81428571 0.82857143 0.84285714 0.85714286 0.87142857 0.88571429 0.9 0.91428571 0.92857143 0.94285714 0.95714286 0.97142857 0.98571429 1 1 1 1 1 1
  arc A22 (-22.2535, -74.7582) -> (-18.107, -75.8692) centre (0, 0) ccw
  spline S11 degree 5 poles (-18.107, -75.8692) (-18.0843, -75.8451) (-18.039, -75.7969) (-17.9712, -75.7244) (-17.8813, -75.6276) (-17.7695, -75.5062) (-17.6583, -75.3845) (-17.5478, -75.2624) (-17.438, -75.14) (-17.3288, -75.0172) (-17.2203, -74.894) (-17.1124, -74.7705) (-17.0053, -74.6467) (-16.8988, -74.5225) (-16.793, -74.3979) (-16.6879, -74.273) (-16.5835, -74.1477) (-16.4798, -74.0221) (-16.3768, -73.8962) (-16.2746, -73.7698) (-16.173, -73.6432) (-16.0722, -73.5162) (-15.9722, -73.3888) (-15.8729, -73.2611) (-15.7743, -73.133) (-15.6765, -73.0046) (-15.5794, -72.8758) (-15.4832, -72.7467) (-15.3877, -72.6172) (-15.293, -72.4874) (-15.1991, -72.3572) (-15.106, -72.2267) (-15.0138, -72.0958) (-14.9224, -71.9645) (-14.8318, -71.8329) (-14.742, -71.701) (-14.6531, -71.5687) (-14.5651, -71.436) (-14.478, -71.303) (-14.3917, -71.1697) (-14.3063, -71.0359) (-14.2219, -70.9018) (-14.1385, -70.7674) (-14.056, -70.6326) (-13.9744, -70.4974) (-13.8938, -70.3618) (-13.8142, -70.2259) (-13.7356, -70.0897) (-13.658, -69.953) (-13.5814, -69.816) (-13.5059, -69.6787) (-13.4316, -69.5409) (-13.3585, -69.4027) (-13.2866, -69.2641) (-13.2159, -69.1252) (-13.1463, -68.9858) (-13.0779, -68.8461) (-13.0105, -68.7061) (-12.9442, -68.5656) (-12.8792, -68.4248) (-12.8159, -68.2835) (-12.7544, -68.1417) (-12.6949, -67.9993) (-12.6374, -67.8564) (-12.5816, -67.713) (-12.5271, -67.5692) (-12.4737, -67.4251) (-12.4211, -67.2808) (-12.37, -67.1362) (-12.3214, -66.991) (-12.277, -66.8447) (-12.2462, -66.7266) (-12.2262, -66.6372) (-12.2145, -66.5773) (-12.2089, -66.5472) knots -1 -1 -1 -1 -1 -1 -0.98571429 -0.97142857 -0.95714286 -0.94285714 -0.92857143 -0.91428571 -0.9 -0.88571429 -0.87142857 -0.85714286 -0.84285714 -0.82857143 -0.81428571 -0.8 -0.78571429 -0.77142857 -0.75714286 -0.74285714 -0.72857143 -0.71428571 -0.7 -0.68571429 -0.67142857 -0.65714286 -0.64285714 -0.62857143 -0.61428571 -0.6 -0.58571429 -0.57142857 -0.55714286 -0.54285714 -0.52857143 -0.51428571 -0.5 -0.48571429 -0.47142857 -0.45714286 -0.44285714 -0.42857143 -0.41428571 -0.4 -0.38571429 -0.37142857 -0.35714286 -0.34285714 -0.32857143 -0.31428571 -0.3 -0.28571429 -0.27142857 -0.25714286 -0.24285714 -0.22857143 -0.21428571 -0.2 -0.18571429 -0.17142857 -0.15714286 -0.14285714 -0.12857143 -0.11428571 -0.1 -0.08571429 -0.07142857 -0.05714286 -0.04285714 -0.02857143 -0.01428571 0 0 0 0 0 0
  line L11 (-12.2089, -66.5472) -> (-12.0953, -65.9278)
  arc A23 (-9.8261, -64.3117) -> (-12.0953, -65.9278) centre (-10.1281, -66.2887) ccw
  arc A24 (-9.8261, -64.3117) -> (-7.1538, -64.6635) centre (0, 0) ccw
  arc A25 (-5.3802, -66.8119) -> (-7.1538, -64.6635) centre (-7.3737, -66.6514) ccw
  line L12 (-5.3802, -66.8119) -> (-5.4307, -67.4396)
  spline S12 degree 5 poles (-5.4307, -67.4396) (-5.4332, -67.47) (-5.4373, -67.531) (-5.4412, -67.6225) (-5.442, -67.7446) (-5.437, -67.8973) (-5.4277, -68.0502) (-5.4157, -68.2031) (-5.4023, -68.3561) (-5.3879, -68.5091) (-5.3725, -68.6621) (-5.3558, -68.815) (-5.3372, -68.968) (-5.3166, -69.1209) (-5.2939, -69.2738) (-5.2693, -69.4267) (-5.243, -69.5795) (-5.2153, -69.7323) (-5.1864, -69.885) (-5.1565, -70.0377) (-5.1253, -70.1903) (-5.093, -70.3428) (-5.0595, -70.4953) (-5.0246, -70.6477) (-4.9885, -70.8) (-4.9511, -70.9522) (-4.9126, -71.1044) (-4.873, -71.2565) (-4.8323, -71.4084) (-4.7906, -71.5603) (-4.7478, -71.7121) (-4.704, -71.8638) (-4.6592, -72.0153) (-4.6134, -72.1668) (-4.5666, -72.3182) (-4.5187, -72.4695) (-4.4699, -72.6206) (-4.4202, -72.7716) (-4.3695, -72.9226) (-4.3179, -73.0734) (-4.2653, -73.224) (-4.2119, -73.3746) (-4.1576, -73.525) (-4.1023, -73.6753) (-4.0462, -73.8255) (-3.9892, -73.9756) (-3.9313, -74.1255) (-3.8726, -74.2752) (-3.8131, -74.4249) (-3.7527, -74.5744) (-3.6914, -74.7237) (-3.6294, -74.873) (-3.5665, -75.022) (-3.5028, -75.171) (-3.4383, -75.3197) (-3.373, -75.4684) (-3.3069, -75.6168) (-3.2401, -75.7652) (-3.1724, -75.9133) (-3.104, -76.0614) (-3.0348, -76.2092) (-2.9648, -76.3569) (-2.8941, -76.5044) (-2.8227, -76.6518) (-2.7505, -76.799) (-2.6775, -76.946) (-2.6038, -77.0929) (-2.5294, -77.2396) (-2.4543, -77.3861) (-2.3784, -77.5325) (-2.3019, -77.6787) (-2.24, -77.7955) (-2.1933, -77.883) (-2.1621, -77.9413) (-2.1464, -77.9705) knots 0 0 0 0 0 0 0.01428571 0.02857143 0.04285714 0.05714286 0.07142857 0.08571429 0.1 0.11428571 0.12857143 0.14285714 0.15714286 0.17142857 0.18571429 0.2 0.21428571 0.22857143 0.24285714 0.25714286 0.27142857 0.28571429 0.3 0.31428571 0.32857143 0.34285714 0.35714286 0.37142857 0.38571429 0.4 0.41428571 0.42857143 0.44285714 0.45714286 0.47142857 0.48571429 0.5 0.51428571 0.52857143 0.54285714 0.55714286 0.57142857 0.58571429 0.6 0.61428571 0.62857143 0.64285714 0.65714286 0.67142857 0.68571429 0.7 0.71428571 0.72857143 0.74285714 0.75714286 0.77142857 0.78571429 0.8 0.81428571 0.82857143 0.84285714 0.85714286 0.87142857 0.88571429 0.9 0.91428571 0.92857143 0.94285714 0.95714286 0.97142857 0.98571429 1 1 1 1 1 1
  arc A26 (-2.1464, -77.9705) -> (2.1464, -77.9705) centre (0, 0) ccw
  spline S13 degree 5 poles (2.1464, -77.9705) (2.1621, -77.9413) (2.1933, -77.883) (2.24, -77.7955) (2.3019, -77.6787) (2.3784, -77.5325) (2.4543, -77.3861) (2.5294, -77.2396) (2.6038, -77.0929) (2.6775, -76.946) (2.7505, -76.799) (2.8227, -76.6518) (2.8941, -76.5044) (2.9648, -76.3569) (3.0348, -76.2092) (3.104, -76.0614) (3.1724, -75.9133) (3.2401, -75.7652) (3.3069, -75.6168) (3.373, -75.4684) (3.4383, -75.3197) (3.5028, -75.171) (3.5665, -75.022) (3.6294, -74.873) (3.6914, -74.7237) (3.7527, -74.5744) (3.8131, -74.4249) (3.8726, -74.2752) (3.9313, -74.1255) (3.9892, -73.9756) (4.0462, -73.8255) (4.1023, -73.6753) (4.1576, -73.525) (4.2119, -73.3746) (4.2653, -73.224) (4.3179, -73.0734) (4.3695, -72.9226) (4.4202, -72.7716) (4.4699, -72.6206) (4.5187, -72.4695) (4.5666, -72.3182) (4.6134, -72.1668) (4.6592, -72.0153) (4.704, -71.8638) (4.7478, -71.7121) (4.7906, -71.5603) (4.8323, -71.4084) (4.873, -71.2565) (4.9126, -71.1044) (4.9511, -70.9522) (4.9885, -70.8) (5.0246, -70.6477) (5.0595, -70.4953) (5.093, -70.3428) (5.1253, -70.1903) (5.1565, -70.0377) (5.1864, -69.885) (5.2153, -69.7323) (5.243, -69.5795) (5.2693, -69.4267) (5.2939, -69.2738) (5.3166, -69.1209) (5.3372, -68.968) (5.3558, -68.815) (5.3725, -68.6621) (5.3879, -68.5091) (5.4023, -68.3561) (5.4157, -68.2031) (5.4277, -68.0502) (5.437, -67.8973) (5.442, -67.7446) (5.4412, -67.6225) (5.4373, -67.531) (5.4332, -67.47) (5.4307, -67.4396) knots -1 -1 -1 -1 -1 -1 -0.98571429 -0.97142857 -0.95714286 -0.94285714 -0.92857143 -0.91428571 -0.9 -0.88571429 -0.87142857 -0.85714286 -0.84285714 -0.82857143 -0.81428571 -0.8 -0.78571429 -0.77142857 -0.75714286 -0.74285714 -0.72857143 -0.71428571 -0.7 -0.68571429 -0.67142857 -0.65714286 -0.64285714 -0.62857143 -0.61428571 -0.6 -0.58571429 -0.57142857 -0.55714286 -0.54285714 -0.52857143 -0.51428571 -0.5 -0.48571429 -0.47142857 -0.45714286 -0.44285714 -0.42857143 -0.41428571 -0.4 -0.38571429 -0.37142857 -0.35714286 -0.34285714 -0.32857143 -0.31428571 -0.3 -0.28571429 -0.27142857 -0.25714286 -0.24285714 -0.22857143 -0.21428571 -0.2 -0.18571429 -0.17142857 -0.15714286 -0.14285714 -0.12857143 -0.11428571 -0.1 -0.08571429 -0.07142857 -0.05714286 -0.04285714 -0.02857143 -0.01428571 0 0 0 0 0 0
  line L13 (5.4307, -67.4396) -> (5.3802, -66.8119)
  arc A27 (7.1538, -64.6635) -> (5.3802, -66.8119) centre (7.3737, -66.6514) ccw
  arc A28 (7.1538, -64.6635) -> (9.8261, -64.3117) centre (0, 0) ccw
  arc A29 (12.0953, -65.9278) -> (9.8261, -64.3117) centre (10.1281, -66.2887) ccw
  line L14 (12.0953, -65.9278) -> (12.2089, -66.5472)
  spline S14 degree 5 poles (12.2089, -66.5472) (12.2145, -66.5773) (12.2262, -66.6372) (12.2462, -66.7266) (12.277, -66.8447) (12.3214, -66.991) (12.37, -67.1362) (12.4211, -67.2808) (12.4737, -67.4251) (12.5271, -67.5692) (12.5816, -67.713) (12.6374, -67.8564) (12.6949, -67.9993) (12.7544, -68.1417) (12.8159, -68.2835) (12.8792, -68.4248) (12.9442, -68.5656) (13.0105, -68.7061) (13.0779, -68.8461) (13.1463, -68.9858) (13.2159, -69.1252) (13.2866, -69.2641) (13.3585, -69.4027) (13.4316, -69.5409) (13.5059, -69.6787) (13.5814, -69.816) (13.658, -69.953) (13.7356, -70.0897) (13.8142, -70.2259) (13.8938, -70.3618) (13.9744, -70.4974) (14.056, -70.6326) (14.1385, -70.7674) (14.2219, -70.9018) (14.3063, -71.0359) (14.3917, -71.1697) (14.478, -71.303) (14.5651, -71.436) (14.6531, -71.5687) (14.742, -71.701) (14.8318, -71.8329) (14.9224, -71.9645) (15.0138, -72.0958) (15.106, -72.2267) (15.1991, -72.3572) (15.293, -72.4874) (15.3877, -72.6172) (15.4832, -72.7467) (15.5794, -72.8758) (15.6765, -73.0046) (15.7743, -73.133) (15.8729, -73.2611) (15.9722, -73.3888) (16.0722, -73.5162) (16.173, -73.6432) (16.2746, -73.7698) (16.3768, -73.8962) (16.4798, -74.0221) (16.5835, -74.1477) (16.6879, -74.273) (16.793, -74.3979) (16.8988, -74.5225) (17.0053, -74.6467) (17.1124, -74.7705) (17.2203, -74.894) (17.3288, -75.0172) (17.438, -75.14) (17.5478, -75.2624) (17.6583, -75.3845) (17.7695, -75.5062) (17.8813, -75.6276) (17.9712, -75.7244) (18.039, -75.7969) (18.0843, -75.8451) (18.107, -75.8692) knots 0 0 0 0 0 0 0.01428571 0.02857143 0.04285714 0.05714286 0.07142857 0.08571429 0.1 0.11428571 0.12857143 0.14285714 0.15714286 0.17142857 0.18571429 0.2 0.21428571 0.22857143 0.24285714 0.25714286 0.27142857 0.28571429 0.3 0.31428571 0.32857143 0.34285714 0.35714286 0.37142857 0.38571429 0.4 0.41428571 0.42857143 0.44285714 0.45714286 0.47142857 0.48571429 0.5 0.51428571 0.52857143 0.54285714 0.55714286 0.57142857 0.58571429 0.6 0.61428571 0.62857143 0.64285714 0.65714286 0.67142857 0.68571429 0.7 0.71428571 0.72857143 0.74285714 0.75714286 0.77142857 0.78571429 0.8 0.81428571 0.82857143 0.84285714 0.85714286 0.87142857 0.88571429 0.9 0.91428571 0.92857143 0.94285714 0.95714286 0.97142857 0.98571429 1 1 1 1 1 1
  arc A30 (18.107, -75.8692) -> (22.2535, -74.7582) centre (0, 0) ccw
  spline S15 degree 5 poles (22.2535, -74.7582) (22.2611, -74.7259) (22.2762, -74.6615) (22.2987, -74.5649) (22.3281, -74.4361) (22.3643, -74.275) (22.3997, -74.1141) (22.4343, -73.9531) (22.4682, -73.7921) (22.5014, -73.6312) (22.5338, -73.4703) (22.5654, -73.3094) (22.5963, -73.1486) (22.6264, -72.9877) (22.6558, -72.827) (22.6843, -72.6663) (22.7121, -72.5056) (22.7391, -72.3449) (22.7653, -72.1844) (22.7907, -72.0239) (22.8153, -71.8634) (22.8391, -71.703) (22.8621, -71.5426) (22.8842, -71.3824) (22.9056, -71.2222) (22.9261, -71.0621) (22.9457, -70.902) (22.9645, -70.7421) (22.9825, -70.5822) (22.9996, -70.4224) (23.0158, -70.2627) (23.0311, -70.1031) (23.0456, -69.9437) (23.0591, -69.7843) (23.0718, -69.625) (23.0835, -69.4659) (23.0944, -69.3069) (23.1043, -69.148) (23.1132, -68.9892) (23.1213, -68.8306) (23.1283, -68.6721) (23.1344, -68.5138) (23.1394, -68.3556) (23.1435, -68.1976) (23.1465, -68.0397) (23.1485, -67.8821) (23.1495, -67.7246) (23.1494, -67.5672) (23.1484, -67.4101) (23.1462, -67.2532) (23.1429, -67.0965) (23.1384, -66.94) (23.1326, -66.7838) (23.1256, -66.6278) (23.1173, -66.4721) (23.1078, -66.3166) (23.0973, -66.1614) (23.0856, -66.0064) (23.0728, -65.8517) (23.0587, -65.6973) (23.0429, -65.5432) (23.0253, -65.3896) (23.0056, -65.2366) (22.9839, -65.084) (22.9605, -64.9319) (22.9358, -64.7802) (22.91, -64.6287) (22.8834, -64.4775) (22.8554, -64.3267) (22.8249, -64.1766) (22.7902, -64.0277) (22.7578, -63.91) (22.7304, -63.8226) (22.7106, -63.7648) (22.7003, -63.736) knots -1 -1 -1 -1 -1 -1 -0.98571429 -0.97142857 -0.95714286 -0.94285714 -0.92857143 -0.91428571 -0.9 -0.88571429 -0.87142857 -0.85714286 -0.84285714 -0.82857143 -0.81428571 -0.8 -0.78571429 -0.77142857 -0.75714286 -0.74285714 -0.72857143 -0.71428571 -0.7 -0.68571429 -0.67142857 -0.65714286 -0.64285714 -0.62857143 -0.61428571 -0.6 -0.58571429 -0.57142857 -0.55714286 -0.54285714 -0.52857143 -0.51428571 -0.5 -0.48571429 -0.47142857 -0.45714286 -0.44285714 -0.42857143 -0.41428571 -0.4 -0.38571429 -0.37142857 -0.35714286 -0.34285714 -0.32857143 -0.31428571 -0.3 -0.28571429 -0.27142857 -0.25714286 -0.24285714 -0.22857143 -0.21428571 -0.2 -0.18571429 -0.17142857 -0.15714286 -0.14285714 -0.12857143 -0.11428571 -0.1 -0.08571429 -0.07142857 -0.05714286 -0.04285714 -0.02857143 -0.01428571 0 0 0 0 0 0
  line L15 (22.7003, -63.736) -> (22.4891, -63.1428)
  arc A31 (23.6462, -60.6086) -> (22.4891, -63.1428) centre (24.3731, -62.4718) ccw
  arc A32 (23.6462, -60.6086) -> (26.1363, -59.5771) centre (0, 0) ccw
  arc A33 (28.7466, -60.5509) -> (26.1363, -59.5771) centre (26.9398, -61.4086) ccw
  line L16 (28.7466, -60.5509) -> (29.0166, -61.1197)
  spline S16 degree 5 poles (29.0166, -61.1197) (29.0297, -61.1474) (29.0566, -61.2022) (29.099, -61.2834) (29.1594, -61.3895) (29.2401, -61.5193) (29.3246, -61.647) (29.4115, -61.7735) (29.4995, -61.8992) (29.5885, -62.0245) (29.6783, -62.1493) (29.7693, -62.2734) (29.8618, -62.3966) (29.9561, -62.5188) (30.0523, -62.6398) (30.15, -62.7599) (30.2492, -62.8791) (30.3496, -62.9976) (30.4509, -63.1154) (30.5532, -63.2327) (30.6565, -63.3493) (30.7607, -63.4652) (30.866, -63.5805) (30.9724, -63.695) (31.0799, -63.8088) (31.1883, -63.922) (31.2978, -64.0345) (31.4081, -64.1464) (31.5193, -64.2576) (31.6314, -64.3683) (31.7443, -64.4784) (31.8581, -64.5879) (31.9727, -64.6967) (32.0881, -64.805) (32.2043, -64.9127) (32.3214, -65.0198) (32.4392, -65.1263) (32.5578, -65.2322) (32.6772, -65.3375) (32.7973, -65.4423) (32.9181, -65.5465) (33.0397, -65.6502) (33.162, -65.7533) (33.2849, -65.8559) (33.4086, -65.9579) (33.533, -66.0593) (33.6581, -66.1602) (33.7838, -66.2606) (33.9102, -66.3604) (34.0373, -66.4596) (34.165, -66.5584) (34.2934, -66.6566) (34.4224, -66.7542) (34.552, -66.8514) (34.6822, -66.948) (34.8131, -67.044) (34.9445, -67.1396) (35.0766, -67.2346) (35.2093, -67.3291) (35.3425, -67.4231) (35.4764, -67.5165) (35.6108, -67.6094) (35.7458, -67.7019) (35.8814, -67.7938) (36.0175, -67.8851) (36.1542, -67.976) (36.2915, -68.0663) (36.4293, -68.1562) (36.5676, -68.2455) (36.7065, -68.3343) (36.8459, -68.4226) (36.9578, -68.4929) (37.042, -68.5453) (37.0983, -68.5802) (37.1264, -68.5976) knots 0 0 0 0 0 0 0.01428571 0.02857143 0.04285714 0.05714286 0.07142857 0.08571429 0.1 0.11428571 0.12857143 0.14285714 0.15714286 0.17142857 0.18571429 0.2 0.21428571 0.22857143 0.24285714 0.25714286 0.27142857 0.28571429 0.3 0.31428571 0.32857143 0.34285714 0.35714286 0.37142857 0.38571429 0.4 0.41428571 0.42857143 0.44285714 0.45714286 0.47142857 0.48571429 0.5 0.51428571 0.52857143 0.54285714 0.55714286 0.57142857 0.58571429 0.6 0.61428571 0.62857143 0.64285714 0.65714286 0.67142857 0.68571429 0.7 0.71428571 0.72857143 0.74285714 0.75714286 0.77142857 0.78571429 0.8 0.81428571 0.82857143 0.84285714 0.85714286 0.87142857 0.88571429 0.9 0.91428571 0.92857143 0.94285714 0.95714286 0.97142857 0.98571429 1 1 1 1 1 1
  arc A34 (37.1264, -68.5976) -> (40.8441, -66.4512) centre (0, 0) ccw